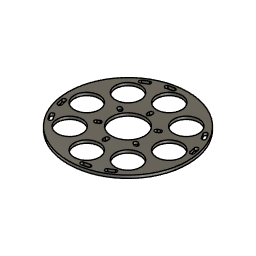
Laser Cut Spool x2 5052 Aluminum 3mm Thick (Autodesk Fusion 360 design; units mm, degrees)
Autodesk Fusion 360 part; units mm, degrees
sketch "Sketch1" plane through (0, 0, 0) normal (0, 0, 1) x (1, 0, 0)
  circle A0 centre (0, 0) radius 100
  circle A1 centre (0, 0) radius 38
  line L0 (0, 0) -> (0, -34.9) construction
  circle A2 centre (0, -34.9) radius 3.1 construction
  circle A3 centre (30.2243, -17.45) radius 3.1
  circle A4 centre (30.2243, 17.45) radius 3.1
  circle A5 centre (0, 34.9) radius 3.1
  circle A6 centre (-30.2243, 17.45) radius 3.1
  circle A7 centre (-30.2243, -17.45) radius 3.1
  circle A8 centre (0, 69) radius 21
  circle A9 centre (0, 0) radius 90
  circle A10 centre (0, 0) radius 48
  line L1 (0, 0) -> (0, 69) construction
  circle A11 centre (0, 0) radius 27.8
  circle A12 centre (0, 0) radius 31.8 construction
  line L2 (-0.8255, -31.9119) -> (-0.8255, -27.7877)
  line L3 (0.8255, -27.7877) -> (0.8255, -31.9119)
  line L4 (24.4776, -13.179) -> (28.0493, -15.2411)
  line L5 (27.2238, -16.6709) -> (23.6521, -14.6088)
  line L6 (23.6521, 14.6088) -> (27.2238, 16.6709)
  line L7 (28.0493, 15.2411) -> (24.4776, 13.179)
  line L8 (-0.8255, 27.7877) -> (-0.8255, 31.9119)
  line L9 (0.8255, 31.9119) -> (0.8255, 27.7877)
  line L10 (-24.4776, 13.179) -> (-28.0493, 15.2411)
  line L11 (-27.2238, 16.6709) -> (-23.6521, 14.6088)
  line L12 (-23.6521, -14.6088) -> (-27.2238, -16.6709)
  line L13 (-28.0493, -15.2411) -> (-24.4776, -13.179)
  circle A13 centre (-48.7904, 48.7904) radius 21
  circle A14 centre (-69, 0) radius 21
  circle A15 centre (-48.7904, -48.7904) radius 21
  circle A16 centre (0, -69) radius 21
  circle A17 centre (48.7904, -48.7904) radius 21
  circle A18 centre (69, 0) radius 21
  circle A19 centre (48.7904, 48.7904) radius 21
  arc A20 (-15.8446, 94.6834) -> (-25.6549, 92.5085) centre (0, 0) ccw
  arc A21 (-25.6549, 92.5085) -> (-24.0515, 86.7267) centre (-24.8532, 89.6176) ccw
  arc A22 (-14.8543, 88.7657) -> (-15.8446, 94.6834) centre (-15.3494, 91.7246) ccw
  line L14 (-24.8532, 89.6176) -> (0, 0) construction
  line L15 (-15.3494, 91.7246) -> (0, 0) construction
  line L16 (-20.7782, 93.7244) -> (0, 0) construction
  arc A23 (-44.3181, 78.332) -> (-47.2727, 83.5541) centre (-45.7954, 80.9431) ccw
  arc A24 (-47.2727, 83.5541) -> (-55.7475, 78.1551) centre (0, 0) ccw
  arc A25 (-55.7475, 78.1551) -> (-52.2633, 73.2704) centre (-54.0054, 75.7127) ccw
  arc A26 (-88.7657, -14.8543) -> (-94.6834, -15.8446) centre (-91.7246, -15.3494) ccw
  arc A27 (-92.5085, -25.6549) -> (-86.7267, -24.0515) centre (-89.6176, -24.8532) ccw
  arc A28 (-94.6834, -15.8446) -> (-92.5085, -25.6549) centre (0, 0) ccw
  arc A29 (-83.5541, -47.2727) -> (-78.1551, -55.7475) centre (0, 0) ccw
  arc A30 (-78.1551, -55.7475) -> (-73.2704, -52.2633) centre (-75.7127, -54.0054) ccw
  arc A31 (-78.332, -44.3181) -> (-83.5541, -47.2727) centre (-80.9431, -45.7954) ccw
  arc A32 (14.8543, -88.7657) -> (15.8446, -94.6834) centre (15.3494, -91.7246) ccw
  arc A33 (25.6549, -92.5085) -> (24.0515, -86.7267) centre (24.8532, -89.6176) ccw
  arc A34 (15.8446, -94.6834) -> (25.6549, -92.5085) centre (0, 0) ccw
  arc A35 (47.2727, -83.5541) -> (55.7475, -78.1551) centre (0, 0) ccw
  arc A36 (55.7475, -78.1551) -> (52.2633, -73.2704) centre (54.0054, -75.7127) ccw
  arc A37 (44.3181, -78.332) -> (47.2727, -83.5541) centre (45.7954, -80.9431) ccw
  arc A38 (88.7657, 14.8543) -> (94.6834, 15.8446) centre (91.7246, 15.3494) ccw
  arc A39 (92.5085, 25.6549) -> (86.7267, 24.0515) centre (89.6176, 24.8532) ccw
  arc A40 (94.6834, 15.8446) -> (92.5085, 25.6549) centre (0, 0) ccw
  arc A41 (83.5541, 47.2727) -> (78.1551, 55.7475) centre (0, 0) ccw
  arc A42 (78.1551, 55.7475) -> (73.2704, 52.2633) centre (75.7127, 54.0054) ccw
  arc A43 (78.332, 44.3181) -> (83.5541, 47.2727) centre (80.9431, 45.7954) ccw
  line L17 (-3.1, -34.9) -> (-3.1, -38.9)
  arc A44 (-3.1, -38.9) -> (3.1, -38.9) centre (0, -38.9) ccw
  line L18 (3.1, -38.9) -> (3.1, -34.9)
  arc A45 (3.1, -34.9) -> (-3.1, -34.9) centre (0, -34.9) ccw
  line L19 (0, -34.9) -> (0, -38.9) construction
  arc A46 (31.7743, -14.7653) -> (28.6743, -20.1347) centre (30.2243, -17.45) ccw
  line L20 (28.6743, -20.1347) -> (32.1384, -22.1347)
  line L21 (35.2384, -16.7653) -> (31.7743, -14.7653)
  arc A47 (32.1384, -22.1347) -> (35.2384, -16.7653) centre (33.6884, -19.45) ccw
  arc A48 (28.6743, 20.1347) -> (31.7743, 14.7653) centre (30.2243, 17.45) ccw
  line L22 (31.7743, 14.7653) -> (35.2384, 16.7653)
  line L23 (32.1384, 22.1347) -> (28.6743, 20.1347)
  arc A49 (35.2384, 16.7653) -> (32.1384, 22.1347) centre (33.6884, 19.45) ccw
  arc A50 (-3.1, 34.9) -> (3.1, 34.9) centre (0, 34.9) ccw
  line L24 (3.1, 34.9) -> (3.1, 38.9)
  line L25 (-3.1, 38.9) -> (-3.1, 34.9)
  arc A51 (3.1, 38.9) -> (-3.1, 38.9) centre (0, 38.9) ccw
  arc A52 (-31.7743, 14.7653) -> (-28.6743, 20.1347) centre (-30.2243, 17.45) ccw
  line L26 (-28.6743, 20.1347) -> (-32.1384, 22.1347)
  line L27 (-35.2384, 16.7653) -> (-31.7743, 14.7653)
  arc A53 (-32.1384, 22.1347) -> (-35.2384, 16.7653) centre (-33.6884, 19.45) ccw
  arc A54 (-28.6743, -20.1347) -> (-31.7743, -14.7653) centre (-30.2243, -17.45) ccw
  line L28 (-31.7743, -14.7653) -> (-35.2384, -16.7653)
  line L29 (-32.1384, -22.1347) -> (-28.6743, -20.1347)
  arc A55 (-35.2384, -16.7653) -> (-32.1384, -22.1347) centre (-33.6884, -19.45) ccw
  dimension "d1" = 200
  dimension "d5" = 76
  dimension "d6" = 6.2
  dimension "d9" = 0
  dimension "d10" = 0
  dimension "d12" = 360
  dimension "d13" = -10
  dimension "d14" = 10
  dimension "d18" = 4
  dimension "d20" = 0.8255
  dimension "d22" = 360
  dimension "d23" = 4
  dimension "d25" = 6
  dimension "d29" = 20
  dimension "d30" = 9.5
  dimension "d32" = 360
  dimension "d35" = 4
  dimension "d37" = 360
  constraint concentric A0 A1
  constraint coincident A0.centre A1.centre
  constraint vertical L0
  constraint coincident L0.end A2.centre
  constraint tangent A1 A2
  constraint tangent A8 A10
  constraint tangent A8 A9
  constraint coincident A8.centre L1.end
  constraint concentric A1 A11
  constraint tangent A6 A12
  constraint coincident A11 L2.end
  constraint vertical L2
  constraint coincident A11 L3.start
  constraint coincident A2 L3.end
  constraint parallel L2 L3
  constraint concentric A0 A20
  constraint tangent A20 A21
  constraint coincident A9 A21.end
  constraint tangent A9 A21
  constraint tangent A9 A22
  constraint coincident A9 A22.start
  constraint tangent A20 A22
  constraint coincident A21.centre L14.start
  constraint coincident A22.centre L15.start
  constraint midpoint A20 L16.start
  constraint coincident A2 L2.start
  constraint vertical L1
  constraint tangent L17 A44
  constraint tangent A44 L18
  constraint parallel L17 L18
  constraint tangent L18 A45
  constraint tangent L17 A45
  constraint parallel L0 L19
  constraint equal A2 A45
  measures "d1" diameter of A0
  measures "d5" diameter of A1
  measures "d6" diameter of A2
  measures "d20" distance of L0 L3
  measures "d23" distance of A0 A20
  measures "d25" angle of L14 L15
  measures "d30" angle of L1 L15
  measures "d35" distance of L0.end A44.centre
extrude "Extrude1" add sketch "Sketch1" along normal blind 4.7498 contours A0 | A1 A3 A4 A11 L4 L7 A46 L21 A48 L22 | A1 A4 A5 A11 L6 L9 A48 L23 A50 L24 | A4 A11 L6 L7 A48 | A1 A3 A11 L3 L5 L18 A45 A46 L20 | A3 A11 L4 L5 A46 | A1 A7 A11 L2 L12 L17 A45 A54 L29 | A1 A5 A6 A11 L8 L11 A50 L25 A52 L26 | A5 A11 L8 L9 A50 | A11 L2 L3 A45 | A6 A11 L10 L11 A52 | A1 A6 A7 A11 L10 L13 A52 L27 A54 L28 | A7 A11 L12 L13 A54 | A8 A9 A10 A19 | A8 A9 A10 A13 | A10 | A9 A10 A18 A19 | A9 A10 A13 A14 | A9 A10 A17 A18 | A9 A10 A14 A15 | A9 A10 A16 A17 | A9 A10 A15 A16
convert_to_sheet_metal "ConvertToSheetMetal1"
sketch "Sketch2" plane through (0, 0, 4.7498) normal (0, 0, 1) x (-1, 0, 0)
  line L0 (-3.1, 34.9) -> (-3.1, 38.9)
  arc A0 (3.1, 38.9) -> (-3.1, 38.9) centre (0, 38.9) ccw
  line L1 (3.1, 38.9) -> (3.1, 34.9)
  arc A1 (-3.1, 34.9) -> (3.1, 34.9) centre (0, 34.9) ccw
  line L2 (28.6743, 20.1347) -> (32.1384, 22.1347)
  arc A2 (35.2384, 16.7653) -> (32.1384, 22.1347) centre (33.6884, 19.45) ccw
  line L3 (35.2384, 16.7653) -> (31.7743, 14.7653)
  arc A3 (28.6743, 20.1347) -> (31.7743, 14.7653) centre (30.2243, 17.45) ccw
  line L4 (31.7743, -14.7653) -> (35.2384, -16.7653)
  arc A4 (32.1384, -22.1347) -> (35.2384, -16.7653) centre (33.6884, -19.45) ccw
  line L5 (32.1384, -22.1347) -> (28.6743, -20.1347)
  arc A5 (31.7743, -14.7653) -> (28.6743, -20.1347) centre (30.2243, -17.45) ccw
  line L6 (3.1, -34.9) -> (3.1, -38.9)
  arc A6 (-3.1, -38.9) -> (3.1, -38.9) centre (0, -38.9) ccw
  line L7 (-3.1, -38.9) -> (-3.1, -34.9)
  arc A7 (3.1, -34.9) -> (-3.1, -34.9) centre (0, -34.9) ccw
  line L8 (-28.6743, -20.1347) -> (-32.1384, -22.1347)
  arc A8 (-35.2384, -16.7653) -> (-32.1384, -22.1347) centre (-33.6884, -19.45) ccw
  line L9 (-35.2384, -16.7653) -> (-31.7743, -14.7653)
  arc A9 (-28.6743, -20.1347) -> (-31.7743, -14.7653) centre (-30.2243, -17.45) ccw
  line L10 (-31.7743, 14.7653) -> (-35.2384, 16.7653)
  arc A10 (-32.1384, 22.1347) -> (-35.2384, 16.7653) centre (-33.6884, 19.45) ccw
  line L11 (-32.1384, 22.1347) -> (-28.6743, 20.1347)
  arc A11 (-31.7743, 14.7653) -> (-28.6743, 20.1347) centre (-30.2243, 17.45) ccw
  circle A12 centre (0, 69) radius 21
  circle A13 centre (-48.7904, -48.7904) radius 21
  arc A14 (-88.7657, -14.8543) -> (-94.6834, -15.8446) centre (-91.7246, -15.3494) ccw
  arc A15 (-88.7657, -14.8543) -> (-86.7267, -24.0515) centre (0, 0) ccw
  arc A16 (-92.5085, -25.6549) -> (-86.7267, -24.0515) centre (-89.6176, -24.8532) ccw
  arc A17 (-94.6834, -15.8446) -> (-92.5085, -25.6549) centre (0, 0) ccw
  arc A18 (44.3181, -78.332) -> (47.2727, -83.5541) centre (45.7954, -80.9431) ccw
  arc A19 (44.3181, -78.332) -> (52.2633, -73.2704) centre (0, 0) ccw
  arc A20 (55.7475, -78.1551) -> (52.2633, -73.2704) centre (54.0054, -75.7127) ccw
  arc A21 (47.2727, -83.5541) -> (55.7475, -78.1551) centre (0, 0) ccw
  circle A22 centre (-48.7904, 48.7904) radius 21
  arc A23 (-44.3181, 78.332) -> (-47.2727, 83.5541) centre (-45.7954, 80.9431) ccw
  arc A24 (-44.3181, 78.332) -> (-52.2633, 73.2704) centre (0, 0) ccw
  arc A25 (-55.7475, 78.1551) -> (-52.2633, 73.2704) centre (-54.0054, 75.7127) ccw
  arc A26 (-47.2727, 83.5541) -> (-55.7475, 78.1551) centre (0, 0) ccw
  arc A27 (14.8543, -88.7657) -> (15.8446, -94.6834) centre (15.3494, -91.7246) ccw
  arc A28 (14.8543, -88.7657) -> (24.0515, -86.7267) centre (0, 0) ccw
  arc A29 (25.6549, -92.5085) -> (24.0515, -86.7267) centre (24.8532, -89.6176) ccw
  arc A30 (15.8446, -94.6834) -> (25.6549, -92.5085) centre (0, 0) ccw
  arc A31 (-78.332, -44.3181) -> (-83.5541, -47.2727) centre (-80.9431, -45.7954) ccw
  arc A32 (-78.332, -44.3181) -> (-73.2704, -52.2633) centre (0, 0) ccw
  arc A33 (-78.1551, -55.7475) -> (-73.2704, -52.2633) centre (-75.7127, -54.0054) ccw
  arc A34 (-83.5541, -47.2727) -> (-78.1551, -55.7475) centre (0, 0) ccw
  arc A35 (-14.8543, 88.7657) -> (-15.8446, 94.6834) centre (-15.3494, 91.7246) ccw
  arc A36 (-14.8543, 88.7657) -> (-24.0515, 86.7267) centre (0, 0) ccw
  arc A37 (-25.6549, 92.5085) -> (-24.0515, 86.7267) centre (-24.8532, 89.6176) ccw
  arc A38 (-15.8446, 94.6834) -> (-25.6549, 92.5085) centre (0, 0) ccw
  circle A39 centre (-69, 0) radius 21
  arc A40 (78.332, 44.3181) -> (83.5541, 47.2727) centre (80.9431, 45.7954) ccw
  arc A41 (78.332, 44.3181) -> (73.2704, 52.2633) centre (0, 0) ccw
  arc A42 (78.1551, 55.7475) -> (73.2704, 52.2633) centre (75.7127, 54.0054) ccw
  arc A43 (83.5541, 47.2727) -> (78.1551, 55.7475) centre (0, 0) ccw
  circle A44 centre (48.7904, -48.7904) radius 21
  circle A45 centre (48.7904, 48.7904) radius 21
  arc A46 (88.7657, 14.8543) -> (94.6834, 15.8446) centre (91.7246, 15.3494) ccw
  arc A47 (88.7657, 14.8543) -> (86.7267, 24.0515) centre (0, 0) ccw
  arc A48 (92.5085, 25.6549) -> (86.7267, 24.0515) centre (89.6176, 24.8532) ccw
  arc A49 (94.6834, 15.8446) -> (92.5085, 25.6549) centre (0, 0) ccw
  circle A50 centre (0, -69) radius 21
  circle A51 centre (69, 0) radius 21
  circle A52 centre (0, 0) radius 100
  circle A53 centre (0, 0) radius 27.8
equation "d20 = 0.065 in / 2"
